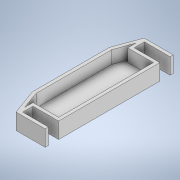
# Autodesk Inventor part: BodyV1
Saved by Autodesk Inventor 2020 (Build 240168000, 168)
## iProperties
Created: 2023-11-25
Part Number: BodyV1
Material: Generic
Document SubType Name: Modeling
Designer: smz3rm
Density: 1 g/cm^3
Appearance: Default
Author: smz3rm
Autodesk Inventor part; units mm, degrees
ref_plane "YZ Plane" through (0, 0, 0) normal (1, 0, 0) x (0, 1, 0)
ref_plane "XZ Plane" through (0, 0, 0) normal (0, 1, 0) x (-1, 0, 0)
ref_plane "XY Plane" through (0, 0, 0) normal (0, 0, 1) x (1, 0, 0)
sketch "Sketch1" plane through (0, 0, 0) normal (0, 1, 0) x (-1, 0, 0)
  line L0 (-38.1, 127) -> (38.1, 127)
  line L1 (38.1, 127) -> (38.1, -127)
  line L2 (38.1, -127) -> (-38.1, -127)
  line L3 (-38.1, -127) -> (-38.1, 127)
  line L4 (-38.1, 127) -> (38.1, -127) construction
  line L5 (38.1, 127) -> (-38.1, -127) construction
  line L6 (19.6103, 127) -> (38.1, 76.2)
  line L7 (53.34, 0) -> (-53.34, 0) projected
  line L8 (19.6103, -127) -> (38.1, -76.2)
  line L9 (12.7, 120.65) -> (-38.1, 120.65)
  line L10 (-38.1, 120.65) -> (-38.1, 100.33)
  line L11 (-38.1, 100.33) -> (12.7, 100.33)
  line L12 (12.7, 100.33) -> (12.7, 120.65)
  line L13 (12.7, -120.65) -> (-38.1, -120.65)
  line L14 (-38.1, -100.33) -> (12.7, -100.33)
  line L15 (12.7, -100.33) -> (12.7, -120.65)
  point P0 (0, 0)
  point P1 (19.6103, -127)
  point P2 (38.1, -76.2)
  point P3 (-38.1, 100.33)
  point P4 (-38.1, -100.33)
  point P5 (-38.1, -120.65)
  dimension "d0" = 76.2
  dimension "d1" = 254
  dimension "d2" = 70
  dimension "d3" = 50.8
  dimension "d6" = 50.8
  dimension "d18" = 20.32
  dimension "d19" = 6.35
  constraints: 30 end point, 6 symmetric about line, 4 parallel, 2 horizontal, 2 midpoint, 2 perpendicular, 2 point on line, 1 collinear
  measures "d0" distance of L1.end L2.end
  measures "d1" distance of L0.end L1.end
  measures "d2" angle of L0 L6
  measures "d3" distance of L0.end L6.end
  measures "d6" distance of L11.end L10.end
  measures "d18" distance of L11.end L9.start
  measures "d19" distance between parallel lines of L0 L9
extrude "Extrusion1" add sketch "Sketch1" along normal blind 6.35 contours L0 L6 L1 L7 L3 L11 L12 L9 | L1 L8 L2 L3 L13 L15 L14 L7
sketch "Sketch4" plane through (0, 6.35, 0) normal (0, 1, 0) x (1, 0, 0)
  line L0 (-38.1, -76.2) -> (-19.6103, -127) projected
  line L1 (-19.6103, -127) -> (38.1, -127) projected
  line L2 (38.1, -127) -> (38.1, -120.65) projected
  line L3 (38.1, -120.65) -> (-12.7, -120.65) projected
  line L4 (-12.7, -120.65) -> (-12.7, -100.33) projected
  line L5 (-12.7, -100.33) -> (38.1, -100.33) projected
  line L6 (38.1, -100.33) -> (38.1, 100.33) projected
  line L7 (38.1, 100.33) -> (-12.7, 100.33) projected
  line L8 (-12.7, 100.33) -> (-12.7, 120.65) projected
  line L9 (-12.7, 120.65) -> (38.1, 120.65) projected
  line L10 (38.1, 120.65) -> (38.1, 127) projected
  line L11 (38.1, 127) -> (-19.6103, 127) projected
  line L12 (-19.6103, 127) -> (-38.1, 76.2) projected
  line L13 (-38.1, 76.2) -> (-38.1, -76.2) projected
  line L14 (-19.05, -109.9733) -> (-31.75, -75.0803)
  line L15 (-31.75, -75.0803) -> (-31.75, 75.0803)
  line L16 (-31.75, 75.0803) -> (-19.05, 109.9733)
  line L17 (-19.05, 109.9733) -> (-19.05, 93.98)
  line L18 (-19.05, 93.98) -> (31.75, 93.98)
  line L19 (31.75, 93.98) -> (31.75, -93.98)
  line L20 (31.75, -93.98) -> (-19.05, -93.98)
  line L21 (-19.05, -93.98) -> (-19.05, -109.9733)
  point P0 (0, 0)
  dimension "d17" = 6.35
  constraints: 16 end point, 7 other
  measures "d17" distance between parallel lines of L0 L14
extrude "Extrusion4" add sketch "Sketch4" along normal blind 25.4
body "Solid1"
